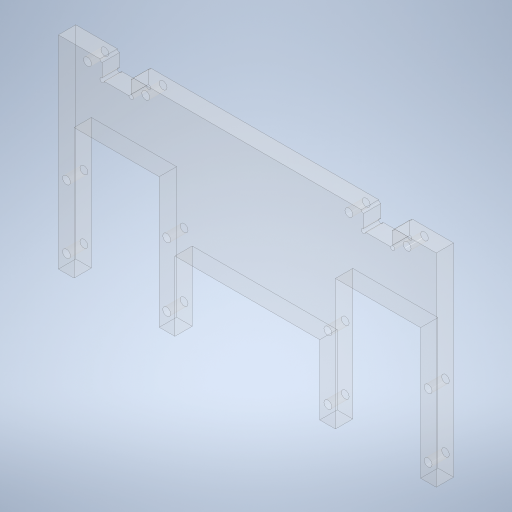
# Autodesk Inventor part: frame_pelvis_to_waist2
Saved by Autodesk Inventor 2024 (Build 280153000, 153)
## iProperties
Created: 2024-09-07
Part Number: frame_pelvis_to_waist2
Material: PMMA 플라스틱
Document SubType Name: Modeling
Designer: jmha0
Density: 1.188 g/cm^3
Appearance: 폴리카보네이트 - 선명
Author: jmha0
Autodesk Inventor part; units mm, degrees
ref_plane "YZ Plane" through (0, 0, 0) normal (1, 0, 0) x (0, 1, 0)
ref_plane "XZ Plane" through (0, 0, 0) normal (0, 1, 0) x (-1, 0, 0)
ref_plane "XY Plane" through (0, 0, 0) normal (0, 0, 1) x (1, 0, 0)
sketch "스케치1" plane through (0, 0, 0) normal (0, 0, 1) x (1, 0, 0)
  arc A0 (90.6223, 135.9255) -> (90.103, 134.2386) centre (93.103, 134.2386) ccw
  line L0 (90.103, 89.9853) -> (90.103, 134.2386)
  arc A1 (90.103, 89.9853) -> (90.6223, 88.2984) centre (93.103, 89.9853) ccw
  line L1 (94.3102, 82.875) -> (90.6223, 88.2984)
  arc A2 (94.3102, 82.875) -> (96.7909, 81.5619) centre (96.7909, 84.5619) ccw
  line L2 (123.6151, 81.5619) -> (96.7909, 81.5619)
  arc A3 (123.6151, 81.5619) -> (126.0959, 82.875) centre (123.6151, 84.5619) ccw
  line L3 (129.7838, 88.2984) -> (126.0959, 82.875)
  arc A4 (129.7838, 88.2984) -> (130.303, 89.9853) centre (127.303, 89.9853) ccw
  line L4 (130.303, 134.2386) -> (130.303, 89.9853)
  arc A5 (130.303, 134.2386) -> (129.7838, 135.9255) centre (127.303, 134.2386) ccw
  line L5 (125.7983, 141.7866) -> (129.7838, 135.9255)
  arc A6 (125.7983, 141.7866) -> (124.1444, 142.6619) centre (124.1444, 140.6619) ccw
  line L6 (117.853, 142.6619) -> (124.1444, 142.6619)
  arc A7 (119.353, 141.1619) -> (117.853, 142.6619) centre (117.853, 141.1619) ccw
  arc A8 (124.703, 136.3119) -> (123.703, 137.3119) centre (123.703, 136.3119) ccw
  line L7 (118.353, 87.1619) -> (102.053, 87.1619)
  line L8 (96.2616, 142.6619) -> (102.553, 142.6619)
  arc A9 (96.2616, 142.6619) -> (94.6078, 141.7866) centre (96.2616, 140.6619) ccw
  line L9 (90.6223, 135.9255) -> (94.6078, 141.7866)
  circle A10 centre (127.503, 133.6619) radius 1.35
  circle A11 centre (127.503, 111.6619) radius 1.35
  circle A12 centre (121.203, 84.3619) radius 1.35
  circle A13 centre (92.903, 133.6619) radius 1.35
  circle A14 centre (92.903, 111.6619) radius 1.35
  circle A15 centre (99.203, 84.3619) radius 1.35
  circle A16 centre (127.503, 89.6619) radius 1.35
  circle A17 centre (92.903, 89.6619) radius 1.35
  arc A18 (180.8223, 135.9255) -> (180.303, 134.2386) centre (183.303, 134.2386) ccw
  line L10 (180.303, 89.9853) -> (180.303, 134.2386)
  arc A19 (180.303, 89.9853) -> (180.8223, 88.2984) centre (183.303, 89.9853) ccw
  line L11 (184.5102, 82.875) -> (180.8223, 88.2984)
  arc A20 (184.5102, 82.875) -> (186.9909, 81.5619) centre (186.9909, 84.5619) ccw
  line L12 (213.8151, 81.5619) -> (186.9909, 81.5619)
  arc A21 (213.8151, 81.5619) -> (216.2959, 82.875) centre (213.8151, 84.5619) ccw
  line L13 (219.9838, 88.2984) -> (216.2959, 82.875)
  arc A22 (219.9838, 88.2984) -> (220.503, 89.9853) centre (217.503, 89.9853) ccw
  line L14 (220.503, 134.2386) -> (220.503, 89.9853)
  arc A23 (220.503, 134.2386) -> (219.9838, 135.9255) centre (217.503, 134.2386) ccw
  line L15 (215.9983, 141.7866) -> (219.9838, 135.9255)
  arc A24 (215.9983, 141.7866) -> (214.3444, 142.6619) centre (214.3444, 140.6619) ccw
  line L16 (208.053, 142.6619) -> (214.3444, 142.6619)
  arc A25 (209.553, 141.1619) -> (208.053, 142.6619) centre (208.053, 141.1619) ccw
  line L17 (211.903, 137.3119) -> (213.903, 137.3119)
  arc A26 (214.903, 136.3119) -> (213.903, 137.3119) centre (213.903, 136.3119) ccw
  line L18 (208.553, 87.1619) -> (192.253, 87.1619)
  arc A27 (186.903, 137.3119) -> (185.903, 136.3119) centre (186.903, 136.3119) ccw
  arc A28 (192.753, 142.6619) -> (191.253, 141.1619) centre (192.753, 141.1619) ccw
  line L19 (186.4616, 142.6619) -> (192.753, 142.6619)
  arc A29 (186.4616, 142.6619) -> (184.8078, 141.7866) centre (186.4616, 140.6619) ccw
  line L20 (180.8223, 135.9255) -> (184.8078, 141.7866)
  circle A30 centre (217.703, 133.6619) radius 1.35
  circle A31 centre (217.703, 111.6619) radius 1.35
  circle A32 centre (211.403, 84.3619) radius 1.35
  circle A33 centre (183.103, 133.6619) radius 1.35
  circle A34 centre (183.103, 111.6619) radius 1.35
  circle A35 centre (189.403, 84.3619) radius 1.35
  circle A36 centre (217.703, 89.6619) radius 1.35
  circle A37 centre (183.103, 89.6619) radius 1.35
  circle A38 centre (200.403, 129.6619) radius 4.5766
  line L21 (95.503, 93.5119) -> (95.503, 136.3119)
  line L22 (124.903, 93.5119) -> (124.903, 136.3119)
  arc A39 (124.903, 136.3119) -> (123.703, 137.5119) centre (123.703, 136.3119) ccw
  line L23 (185.703, 93.5119) -> (185.703, 136.3119)
  arc A40 (186.903, 137.5119) -> (185.703, 136.3119) centre (186.903, 136.3119) ccw
  line L24 (215.103, 93.5119) -> (215.103, 136.3119)
  arc A41 (215.103, 136.3119) -> (213.903, 137.5119) centre (213.903, 136.3119) ccw
  line L25 (213.903, 137.5119) -> (211.903, 137.5119)
  line L26 (90.103, 129.6619) -> (90.103, 105.6619)
  line L27 (90.103, 105.6619) -> (220.503, 105.6619)
  line L28 (220.503, 105.6619) -> (220.503, 129.6619)
  line L29 (220.503, 129.6619) -> (90.103, 129.6619)
  line L30 (90.103, 129.6619) -> (90.103, 105.6619)
  line L31 (90.103, 129.6619) -> (220.503, 129.6619)
  line L32 (220.503, 129.6619) -> (220.503, 175.6619)
  line L33 (220.503, 175.6619) -> (90.103, 175.6619)
  line L34 (90.103, 175.6619) -> (90.103, 129.6619)
  line L35 (95.503, 140.6619) -> (215.103, 140.6619)
  line L36 (215.103, 140.6619) -> (215.103, 129.6619)
  line L37 (185.703, 129.6619) -> (185.703, 140.6619)
  line L38 (124.903, 129.6619) -> (124.903, 140.6619)
  line L39 (95.503, 129.6619) -> (95.503, 140.6619)
  line L40 (95.503, 140.6619) -> (95.503, 150.6619)
  line L41 (124.903, 140.6619) -> (124.903, 150.6619)
  line L42 (124.903, 150.6619) -> (95.503, 150.6619)
  line L43 (185.703, 140.6619) -> (185.703, 150.6619)
  line L44 (185.703, 150.6619) -> (215.103, 150.6619)
  line L45 (215.103, 150.6619) -> (215.103, 140.6619)
  point P0 (110.203, 129.6619)
  point P1 (90.103, 134.2386)
  point P2 (95.503, 105.6619)
  point P3 (124.903, 105.6619)
  point P4 (130.303, 105.6619)
  point P5 (130.303, 129.6619)
  point P6 (180.303, 129.6619)
  point P7 (180.303, 105.6619)
  point P8 (185.703, 105.6619)
  point P9 (215.103, 129.6619)
  point P10 (215.103, 105.6619)
  dimension "d18" = 24
  dimension "d19" = 46
  dimension "d33" = 10
  constraints: 92 end point, 50 point on circle, 42 centre point, 17 point on line, 7 perpendicular, 6 parallel, 2 vertical, 1 other
  measures "d18" distance of L26.start L26.end
  measures "d19" distance of L32.end L28.end
  measures "d33" distance of L35.start L40.end
extrude "돌출2" add sketch "스케치1" along normal blind 6 contours L9 A9 L40 L39 L21 L29 L0 A0 | A0 L34 L33 L32 A23 L15 A24 L45 L44 L43 A29 L20 L35 L5 A6 L41 L42 L40 A9 L9 | L29 L21 L27 L0 | L29 L4 L27 L22 | L22 L38 L35 L5 A5 L4 L29 | L14 L29 L24 L36 L45 A24 L15 A23 | L41 A6 L5 L35 | L4 A5 L5 L35 L20 A18 L10 L29 | L14 L27 L24 L29 | L29 L23 L27 L10 | L10 A18 L20 L35 L37 L23 L29 | L20 A29 L43 L35
sketch "스케치2" plane through (0, 0, 6) normal (0, 0, 1) x (1, 0, 0)
  line L0 (220.503, 175.6619) -> (90.103, 175.6619) projected
  line L1 (90.103, 175.6619) -> (90.103, 105.6619) projected
  line L2 (90.103, 105.6619) -> (95.503, 105.6619) projected
  line L3 (95.503, 105.6619) -> (95.503, 150.6619) projected
  line L4 (124.903, 150.6619) -> (124.903, 105.6619) projected
  line L5 (124.903, 105.6619) -> (130.303, 105.6619) projected
  line L6 (130.303, 105.6619) -> (130.303, 129.6619) projected
  line L7 (130.303, 129.6619) -> (180.303, 129.6619) projected
  line L8 (180.303, 129.6619) -> (180.303, 105.6619) projected
  line L9 (180.303, 105.6619) -> (185.703, 105.6619) projected
  line L10 (185.703, 105.6619) -> (185.703, 150.6619) projected
  line L11 (215.103, 150.6619) -> (215.103, 105.6619) projected
  line L12 (215.103, 105.6619) -> (220.503, 105.6619) projected
  line L13 (220.503, 105.6619) -> (220.503, 175.6619) projected
  circle A0 centre (127.503, 111.6619) radius 1.35 projected
  circle A1 centre (217.703, 111.6619) radius 1.35 projected
  circle A2 centre (127.503, 133.6619) radius 1.35 projected
  circle A3 centre (183.103, 133.6619) radius 1.35 projected
  circle A4 centre (183.103, 111.6619) radius 1.35 projected
  circle A5 centre (217.703, 133.6619) radius 1.35 projected
  circle A6 centre (92.903, 133.6619) radius 1.35 projected
  circle A7 centre (92.903, 111.6619) radius 1.35 projected
  line L14 (90.103, 175.6619) -> (220.503, 175.6619)
  line L15 (220.503, 175.6619) -> (220.503, 169.6619)
  line L16 (220.503, 169.6619) -> (90.103, 169.6619)
  line L17 (90.103, 169.6619) -> (90.103, 175.6619)
  line L18 (90.103, 172.6619) -> (100.153, 172.6619)
  line L19 (100.153, 172.6619) -> (120.253, 172.6619)
  line L20 (220.503, 172.6619) -> (210.453, 172.6619)
  line L21 (210.453, 172.6619) -> (190.353, 172.6619)
  circle A8 centre (100.153, 172.6619) radius 1.35
  circle A9 centre (120.253, 172.6619) radius 1.35
  circle A10 centre (190.353, 172.6619) radius 1.35
  circle A11 centre (210.453, 172.6619) radius 1.35
  line L22 (95.503, 150.6619) -> (124.903, 150.6619) projected
  line L23 (185.703, 150.6619) -> (215.103, 150.6619) projected
  point P0 (0, 0)
  dimension "d22" = 6
  dimension "d23" = 10.05
  dimension "d24" = 20.1
  dimension "d25" = 10.05
  dimension "d26" = 20.1
  dimension "d27" = 2.7
  dimension "d28" = 2.7
  dimension "d29" = 2.7
  dimension "d30" = 2.7
  constraints: 16 end point, 4 centre point, 4 coincident, 3 horizontal, 3 point on line, 2 midpoint, 2 parallel, 1 perpendicular
  measures "d22" distance of L14.end L15.end
  measures "d23" distance of L18.start L18.end
  measures "d24" distance of L18.end L19.end
  measures "d25" distance of L20.start L20.end
  measures "d26" distance of L20.end L21.end
  measures "d27" diameter of A8
  measures "d28" diameter of A9
  measures "d29" diameter of A10
  measures "d30" diameter of A11
extrude "돌출3" cut sketch "스케치2" against normal blind 6 contours A9 | A8 L19 L18 | L18 L19 A8 | A10 | A11 L21 L20 | L20 L21 A11
sketch "스케치3" plane through (0, 0, 6) normal (0, 0, 1) x (1, 0, 0)
  circle A0 centre (120.253, 172.6619) radius 1.35 projected
  circle A1 centre (190.353, 172.6619) radius 1.35 projected
  circle A2 centre (100.153, 172.6619) radius 1.35 projected
  circle A3 centre (210.453, 172.6619) radius 1.35 projected
  line L0 (95.503, 150.6619) -> (124.903, 150.6619) projected
  line L1 (124.903, 150.6619) -> (124.903, 105.6619) projected
  line L2 (124.903, 105.6619) -> (130.303, 105.6619) projected
  line L3 (130.303, 105.6619) -> (130.303, 129.6619) projected
  line L4 (130.303, 129.6619) -> (180.303, 129.6619) projected
  line L5 (180.303, 129.6619) -> (180.303, 105.6619) projected
  line L6 (180.303, 105.6619) -> (185.703, 105.6619) projected
  line L7 (185.703, 105.6619) -> (185.703, 150.6619) projected
  line L8 (185.703, 150.6619) -> (215.103, 150.6619) projected
  line L9 (215.103, 150.6619) -> (215.103, 105.6619) projected
  line L10 (215.103, 105.6619) -> (220.503, 105.6619) projected
  line L11 (220.503, 105.6619) -> (220.503, 175.6619) projected
  line L12 (220.503, 175.6619) -> (90.103, 175.6619) projected
  line L13 (90.103, 175.6619) -> (90.103, 105.6619) projected
  line L14 (90.103, 105.6619) -> (95.503, 105.6619) projected
  line L15 (95.503, 105.6619) -> (95.503, 150.6619) projected
  circle A4 centre (127.503, 111.6619) radius 1.35 projected
  circle A5 centre (92.903, 111.6619) radius 1.35 projected
  circle A6 centre (92.903, 133.6619) radius 1.35 projected
  circle A7 centre (217.703, 111.6619) radius 1.35 projected
  circle A8 centre (217.703, 133.6619) radius 1.35 projected
  circle A9 centre (183.103, 111.6619) radius 1.35 projected
  circle A10 centre (183.103, 133.6619) radius 1.35 projected
  circle A11 centre (127.503, 133.6619) radius 1.35 projected
  line L16 (105.203, 169.6619) -> (105.203, 175.6619)
  line L17 (105.203, 175.6619) -> (115.203, 175.6619)
  line L18 (115.203, 175.6619) -> (115.203, 169.6619)
  line L19 (115.203, 169.6619) -> (105.203, 169.6619)
  line L20 (105.203, 169.6619) -> (115.203, 175.6619) construction
  line L21 (105.203, 175.6619) -> (115.203, 169.6619) construction
  line L22 (205.403, 169.6619) -> (205.403, 175.6619)
  line L23 (205.403, 175.6619) -> (195.403, 175.6619)
  line L24 (195.403, 175.6619) -> (195.403, 169.6619)
  line L25 (195.403, 169.6619) -> (205.403, 169.6619)
  line L26 (205.403, 169.6619) -> (195.403, 175.6619) construction
  line L27 (205.403, 175.6619) -> (195.403, 169.6619) construction
  point P0 (0, 0)
  point P1 (110.203, 172.6619)
  point P2 (200.403, 172.6619)
  dimension "d34" = 10
  dimension "d35" = 10
  constraints: 24 end point, 4 midpoint, 4 parallel, 4 perpendicular
  measures "d34" distance of L16.end L17.end
  measures "d35" distance of L23.end L22.end
extrude "돌출4" cut sketch "스케치3" against normal blind 6 contours L12 L18 L19 L16 | L12 L22 L25 L24
sketch "스케치4" plane through (0, 0, 6) normal (0, 0, 1) x (1, 0, 0)
  line L0 (195.403, 169.6619) -> (195.403, 175.6619) projected
  line L1 (195.403, 175.6619) -> (115.203, 175.6619) projected
  line L2 (115.203, 175.6619) -> (115.203, 169.6619) projected
  line L3 (115.203, 169.6619) -> (105.203, 169.6619) projected
  line L4 (105.203, 169.6619) -> (105.203, 175.6619) projected
  line L5 (105.203, 175.6619) -> (90.103, 175.6619) projected
  line L6 (90.103, 175.6619) -> (90.103, 105.6619) projected
  line L7 (90.103, 105.6619) -> (95.503, 105.6619) projected
  line L8 (95.503, 105.6619) -> (95.503, 150.6619) projected
  line L9 (95.503, 150.6619) -> (124.903, 150.6619) projected
  line L10 (124.903, 150.6619) -> (124.903, 105.6619) projected
  line L11 (124.903, 105.6619) -> (130.303, 105.6619) projected
  line L12 (130.303, 105.6619) -> (130.303, 129.6619) projected
  line L13 (130.303, 129.6619) -> (180.303, 129.6619) projected
  line L14 (180.303, 129.6619) -> (180.303, 105.6619) projected
  line L15 (180.303, 105.6619) -> (185.703, 105.6619) projected
  line L16 (185.703, 105.6619) -> (185.703, 150.6619) projected
  line L17 (185.703, 150.6619) -> (215.103, 150.6619) projected
  line L18 (215.103, 150.6619) -> (215.103, 105.6619) projected
  line L19 (215.103, 105.6619) -> (220.503, 105.6619) projected
  line L20 (220.503, 105.6619) -> (220.503, 175.6619) projected
  line L21 (220.503, 175.6619) -> (205.403, 175.6619) projected
  line L22 (205.403, 175.6619) -> (205.403, 169.6619) projected
  line L23 (205.403, 169.6619) -> (195.403, 169.6619) projected
  circle A0 centre (120.253, 172.6619) radius 1.35 projected
  circle A1 centre (190.353, 172.6619) radius 1.35 projected
  circle A2 centre (100.153, 172.6619) radius 1.35 projected
  circle A3 centre (210.453, 172.6619) radius 1.35 projected
  circle A4 centre (127.503, 111.6619) radius 1.35 projected
  circle A5 centre (92.903, 111.6619) radius 1.35 projected
  circle A6 centre (92.903, 133.6619) radius 1.35 projected
  circle A7 centre (217.703, 111.6619) radius 1.35 projected
  circle A8 centre (217.703, 133.6619) radius 1.35 projected
  circle A9 centre (183.103, 111.6619) radius 1.35 projected
  circle A10 centre (183.103, 133.6619) radius 1.35 projected
  circle A11 centre (127.503, 133.6619) radius 1.35 projected
  circle A12 centre (105.203, 175.6619) radius 0.75
  circle A13 centre (105.203, 169.6619) radius 0.75
  circle A14 centre (115.203, 169.6619) radius 0.75
  circle A15 centre (115.203, 175.6619) radius 0.75
  line L24 (195.403, 175.6619) -> (115.203, 175.6619) projected
  circle A16 centre (195.403, 175.6619) radius 0.75
  circle A17 centre (205.403, 175.6619) radius 0.75
  line L25 (205.403, 175.6619) -> (205.403, 169.6619) projected
  circle A18 centre (205.403, 169.6619) radius 0.75
  circle A19 centre (195.403, 169.6619) radius 0.75
  point P0 (0, 0)
  dimension "d38" = 1.5
  dimension "d39" = 1.5
  dimension "d40" = 1.5
  dimension "d41" = 1.5
  dimension "d42" = 1.5
  dimension "d43" = 1.5
  dimension "d44" = 1.5
  dimension "d45" = 1.5
  constraints: 8 centre point, 8 coincident
  measures "d38" diameter of A12
  measures "d39" diameter of A13
  measures "d40" diameter of A14
  measures "d41" diameter of A15
  measures "d42" diameter of A16
  measures "d43" diameter of A17
  measures "d44" diameter of A18
  measures "d45" diameter of A19
extrude "돌출5" cut sketch "스케치4" against normal blind 6 contours L23 A19 L0 | L0 A19 L23 | A16 L1 L0 | L0 L1 A16 | A18 L22 L23 | L23 L22 A18 | A15 L2 L1 | L1 L2 A15 | A17 L21 L22 | L22 L21 A17 | A14 L3 L2 | L2 L3 A14 | A13 L4 L3 | L3 L4 A13 | A12 L5 L4 | L4 L5 A12
